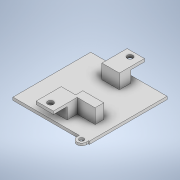
# Autodesk Inventor part: uchwyt2
Saved by Autodesk Inventor 2020.3 (Build 243373000, 373)
## iProperties
Created: 2021-02-11
Part Number: uchwyt2
Material: Ogólny
Document SubType Name: Modeling
Designer: sitar
Density: 1 g/cm^3
Appearance: Domyślna
Author: sitar
Autodesk Inventor part; units mm, degrees
ref_plane "YZ Plane" through (0, 0, 0) normal (1, 0, 0) x (0, 1, 0)
ref_plane "XZ Plane" through (0, 0, 0) normal (0, 1, 0) x (-1, 0, 0)
ref_plane "XY Plane" through (0, 0, 0) normal (0, 0, 1) x (1, 0, 0)
sketch "Szkic1" plane through (0, 0, 0) normal (0, 1, 0) x (-1, 0, 0)
  line L0 (26.7, -27.1) -> (-26.7, -27.1)
  line L1 (-26.7, -27.1) -> (-26.7, 27.1)
  line L2 (-26.7, 27.1) -> (26.7, 27.1)
  line L3 (26.7, 27.1) -> (26.7, -27.1)
  line L4 (26.7, -27.1) -> (-26.7, 27.1) construction
  line L5 (-26.7, -27.1) -> (26.7, 27.1) construction
  point P0 (0, 0)
  dimension "d0" = 53.4
  dimension "d1" = 54.2
  constraints: 12 end point, 2 midpoint, 2 parallel, 1 horizontal, 1 perpendicular
  measures "d0" distance of L1.end L2.end
  measures "d1" distance of L0.end L1.end
extrude "Wyciągnięcie proste1" add sketch "Szkic1" along normal blind 1.6
sketch "Szkic11" plane through (0, 1.6, 0) normal (0, 1, 0) x (1, 0, 0)
  line L0 (-26.7, -27.1) -> (26.7, -27.1) projected
  line L1 (26.7, -27.1) -> (25.9, -27.1)
  line L2 (25.9, -27.1) -> (19.5, -27.1)
  line L3 (19.5, -27.1) -> (19.5, -28.7)
  line L4 (19.5, -28.7) -> (25.9, -28.7)
  line L5 (25.9, -28.7) -> (25.9, -27.1)
  arc A0 (19.5, -28.7) -> (25.9, -28.7) centre (22.7, -28.7) ccw
  point P0 (0, 0)
  dimension "d37" = 0.8
  dimension "d38" = 6.4
  dimension "d39" = 1.6
  dimension "d40" = 3.2
  constraints: 10 end point, 2 parallel, 2 point on circle, 1 centre point, 1 horizontal, 1 perpendicular, 1 point on line
  measures "d37" distance of L0.end L1.end
  measures "d38" distance of L4.end L3.end
  measures "d39" distance of L3.end L2.end
  measures "d40" radius of A0
extrude "Wyciągnięcie proste10" add sketch "Szkic11" against normal blind 1.6
sketch "Szkic12" plane through (0, 1.6, 0) normal (0, 1, 0) x (1, 0, 0)
  arc A0 (19.5, -28.7) -> (25.9, -28.7) centre (22.7, -28.7) ccw projected
  circle A1 centre (22.7, -28.7) radius 1.6
  point P0 (0, 0)
  dimension "d43" = 3.2
  constraints: 1 centre point, 1 coincident
  measures "d43" diameter of A1
extrude "Wyciągnięcie proste11" cut sketch "Szkic12" against normal through all
sketch "Szkic24" plane through (0, 1.6, 0) normal (0, 1, 0) x (1, 0, 0)
  line L0 (11.2, -12.1) -> (11.2, -27.1)
  line L1 (-26.7, -27.1) -> (19.5, -27.1) projected
  line L2 (11.2, -12.1) -> (26.2, -12.1) construction
  line L3 (11.2, -12.1) -> (26.7, -12.1)
  line L4 (26.7, -27.1) -> (26.7, 27.1) projected
  line L5 (11.2, -12.1) -> (26.7, -12.1) construction
  line L6 (4.8, -9.9) -> (17.6, -9.9)
  line L7 (17.6, -9.9) -> (17.6, -14.3)
  line L8 (17.6, -14.3) -> (4.8, -14.3)
  line L9 (4.8, -14.3) -> (4.8, -9.9)
  line L10 (4.8, -9.9) -> (17.6, -14.3) construction
  line L11 (17.6, -9.9) -> (4.8, -14.3) construction
  point P0 (0, 0)
  dimension "d104" = 15
  dimension "d105" = 90
  dimension "d106" = 15.5
  dimension "d107" = 0
  dimension "d108" = 12.8
  dimension "d109" = 4.4
  constraints: 20 end point, 3 horizontal, 3 perpendicular, 2 equal length, 2 midpoint, 2 parallel, 2 point on line
  measures "d104" distance of L0.start L0.end
  measures "d105" angle of L0 L2
  measures "d106" distance of L0.start L3.end
  measures "d107" distance between parallel lines of L3 L5
  measures "d108" distance of L7.end L8.end
  measures "d109" distance of L6.end L7.end
extrude "Wyciągnięcie proste22" cut sketch "Szkic24" against normal through all
sketch "Szkic33" plane through (0, 1.6, 0) normal (0, 1, 0) x (1, 0, 0)
  line L0 (4.8, -14.3) -> (17.6, -14.3) projected
  line L1 (4, 4) -> (4, 25.6) projected
  line L2 (17.6, -14.3) -> (4, -14.3)
  line L3 (4, -14.3) -> (4, -15.1)
  line L4 (4, -15.1) -> (17.6, -15.1)
  line L5 (17.6, -15.1) -> (17.6, -14.3)
  line L6 (4, -15.1) -> (4.8, -15.1)
  line L7 (4.8, -15.1) -> (4.8, -9.1)
  line L8 (4.8, -9.1) -> (4, -9.1)
  line L9 (4, -9.1) -> (4, -15.1)
  line L10 (17.6, -15.1) -> (18.4, -15.1)
  line L11 (18.4, -15.1) -> (18.4, -9.1)
  line L12 (18.4, -9.1) -> (17.6, -9.1)
  line L13 (17.6, -9.1) -> (17.6, -15.1)
  point P0 (0, 0)
  point P1 (4, -21.6)
  point P2 (4, -10)
  point P3 (17.6, -14.3)
  point P4 (4, -10)
  dimension "d139" = 0.8
  dimension "d140" = 6
  dimension "d141" = 0.8
  constraints: 24 end point, 6 parallel, 3 horizontal, 3 perpendicular, 2 point on line
  measures "d139" distance of L3.end L2.end
  measures "d140" distance of L7.end L6.end
  measures "d141" distance of L12.end L11.end
extrude "Wyciągnięcie proste30" add sketch "Szkic33" along normal blind 10
sketch "Szkic34" plane through (0, 1.6, 0) normal (0, 1, 0) x (1, 0, 0)
  line L0 (17.6, -9.9) -> (4.8, -9.9) projected
  line L1 (4.8, -14.3) -> (4.8, -9.1) projected
  line L2 (17.6, -9.9) -> (4.8, -9.9)
  line L3 (4.8, -9.9) -> (4.8, -9.1)
  line L4 (4.8, -9.1) -> (17.6, -9.1)
  line L5 (17.6, -9.1) -> (17.6, -9.9)
  point P0 (0, 0)
  constraints: 8 end point, 2 parallel, 1 horizontal, 1 perpendicular
extrude "Wyciągnięcie proste31" add sketch "Szkic34" along normal blind 2
sketch "Szkic35" plane through (0, 11.6, 0) normal (0, 1, 0) x (1, 0, 0)
  line L0 (4.8, -9.1) -> (4, -9.1) projected
  line L1 (18.4, -15.1) -> (4, -15.1)
  line L2 (4, -15.1) -> (4, -9.1)
  line L3 (4, -9.1) -> (18.4, -9.1)
  line L4 (18.4, -9.1) -> (18.4, -15.1)
  point P0 (0, 0)
  point P1 (4.8, -9.1)
  constraints: 8 end point, 2 parallel, 1 horizontal, 1 perpendicular
extrude "Wyciągnięcie proste32" add sketch "Szkic35" against normal blind 0.8
sketch "Szkic49" plane through (26.7, 0, 27.1) normal (1, 0, 0) x (0, 0, -1)
  line L0 (54.2, 0) -> (54.2, 1.6) projected
  line L1 (0, 0) -> (54.2, 0)
  line L2 (54.2, 0) -> (54.2, 1.6)
  line L3 (54.2, 1.6) -> (0, 1.6)
  line L4 (0, 1.6) -> (0, 0)
  point P0 (27.1, 0)
  constraints: 8 end point, 2 parallel, 1 horizontal, 1 perpendicular
extrude "Wyciągnięcie proste41" cut sketch "Szkic49" against normal blind 0.3
sketch "Szkic50" plane through (-26.7, 0, -27.1) normal (-1, 0, 0) x (0, 0, 1)
  line L0 (0, 1.6) -> (0, 0) projected
  line L1 (0, 0) -> (54.2, 0) projected
  line L2 (0, 1.6) -> (54.2, 1.6)
  line L3 (54.2, 1.6) -> (54.2, 0)
  line L4 (54.2, 0) -> (0, 0)
  line L5 (0, 0) -> (0, 1.6)
  point P0 (27.1, 0)
  constraints: 8 end point, 2 parallel, 1 horizontal, 1 perpendicular
extrude "Wyciągnięcie proste42" cut sketch "Szkic50" against normal blind 0.3
sketch "Szkic57" plane through (0, 0, 0) normal (0, -1, 0) x (1, 0, 0)
  line L0 (-26.4, -27.1) -> (-26.4, 27.1) projected
  line L1 (-26.4, 27.1) -> (26.4, 27.1)
  line L2 (26.4, 27.1) -> (26.4, -27.1)
  line L3 (26.4, -27.1) -> (-26.4, -27.1)
  line L4 (-26.4, -27.1) -> (-26.4, 27.1)
  line L5 (4.8, 14.3) -> (17.6, 14.3) projected
  line L6 (4.8, 9.9) -> (17.6, 9.9) projected
  line L7 (4.8, 14.3) -> (17.6, 14.3)
  line L8 (17.6, 14.3) -> (17.6, 9.9)
  line L9 (17.6, 9.9) -> (4.8, 9.9)
  line L10 (4.8, 9.9) -> (4.8, 14.3)
  point P0 (0, 0)
  point P1 (17.6, 14.3)
  constraints: 16 end point, 4 parallel, 2 horizontal, 2 perpendicular
extrude "Wyciągnięcie proste48" add sketch "Szkic57" along normal blind 0.4
sketch "Szkic62" plane through (26.4, 1.6, -27.1) normal (0, 0, -1) x (-1, 0, 0)
  line L0 (52.8, 0) -> (52.8, -2) projected
  line L1 (52.8, -2) -> (0, -2)
  line L2 (0, -2) -> (0, 0)
  line L3 (0, 0) -> (52.8, 0)
  line L4 (52.8, 0) -> (52.8, -2)
  point P0 (26.4, -1.6)
  constraints: 8 end point, 2 parallel, 1 horizontal, 1 perpendicular
extrude "Wyciągnięcie proste52" cut sketch "Szkic62" against normal blind 0.4
sketch "Szkic63" plane through (0, 1.6, 0) normal (0, 1, 0) x (1, 0, 0)
  line L0 (0, 0) -> (0, 27.5)
  line L1 (0, 0) -> (27.5, 0) construction
  circle A0 centre (0, 27.5) radius 2
  line L2 (0, 0) -> (0, -27.5)
  line L3 (0, 0) -> (27.5, 0) construction
  circle A1 centre (0, -27.5) radius 2
  dimension "d235" = 27.5
  dimension "d236" = 90
  dimension "d237" = 4
  dimension "d238" = 27.5
  dimension "d239" = 90
  dimension "d240" = 4
  constraints: 8 end point, 2 centre point, 2 coincident, 2 horizontal, 2 perpendicular, 2 vertical
  measures "d235" distance of L0.start L0.end
  measures "d236" angle of L1 L0
  measures "d237" diameter of A0
  measures "d238" distance of L0.start L2.end
  measures "d239" angle of L2 L3
  measures "d240" diameter of A1
sketch "Szkic64" plane through (0, 1.6, 0) normal (0, 1, 0) x (1, 0, 0)
  line L0 (26.4, 26.7) -> (-26.4, 26.7) projected
  line L1 (0, 26.7) -> (0, 25.1)
  line L2 (0, 25.1) -> (-4, 25.1)
  line L3 (-4, 25.1) -> (-4, 18.7)
  line L4 (-4, 18.7) -> (0, 18.7)
  line L5 (0, 18.7) -> (0, 25.1)
  point P0 (0, 0)
  dimension "d241" = 1.6
  dimension "d242" = 4
  dimension "d243" = 6.4
  constraints: 10 end point, 2 parallel, 1 horizontal, 1 midpoint, 1 perpendicular, 1 vertical
  measures "d241" distance of L1.start L1.end
  measures "d242" distance of L4.end L3.end
  measures "d243" distance of L3.end L2.end
extrude "Wyciągnięcie proste53" add sketch "Szkic64" along normal blind 8
mirror "Odbij11" about plane through (0, 0, 0) normal (1, 0, 0) of "Wyciągnięcie proste53"
sketch "Szkic65" plane through (0, 9.6, 0) normal (0, 1, 0) x (1, 0, 0)
  line L0 (-4, 25.1) -> (4, 25.1) projected
  line L1 (-4, 25.1) -> (4, 25.1)
  line L2 (4, 25.1) -> (4, 31.5)
  line L3 (4, 31.5) -> (-4, 31.5)
  line L4 (-4, 31.5) -> (-4, 25.1)
  point P0 (0, 0)
  dimension "d246" = 6.4
  constraints: 8 end point, 2 parallel, 1 horizontal, 1 perpendicular
  measures "d246" distance of L2.end L1.end
extrude "Wyciągnięcie proste54" add sketch "Szkic65" along normal blind 2
mirror "Odbij12" about plane through (0, 0, 0) normal (0, 0, 1) of "Wyciągnięcie proste53", "Odbij11", "Wyciągnięcie proste54"
extrude "Wyciągnięcie proste55" cut sketch "Szkic63" along normal through all
sketch "Szkic66" plane through (0, 9.6, 0) normal (0, 1, 0) x (1, 0, 0)
  line L0 (-4, 18.7) -> (-4, 25.1) projected
  line L1 (-4, 25.1) -> (4, 25.1) projected
  line L2 (-4, 18.7) -> (4, 18.7)
  line L3 (4, 18.7) -> (4, 25.1)
  line L4 (4, 25.1) -> (-4, 25.1)
  line L5 (-4, 25.1) -> (-4, 18.7)
  line L6 (-4, -25.1) -> (-4, -18.7) projected
  line L7 (-4, -25.1) -> (4, -25.1) projected
  line L8 (-4, -18.7) -> (4, -18.7)
  line L9 (4, -18.7) -> (4, -25.1)
  line L10 (4, -25.1) -> (-4, -25.1)
  line L11 (-4, -25.1) -> (-4, -18.7)
  point P0 (0, 0)
  constraints: 16 end point, 4 parallel, 2 horizontal, 2 perpendicular
extrude "Wyciągnięcie proste56" add sketch "Szkic66" along normal blind 2
sketch "Szkic67" plane through (4, 1.6, -25.1) normal (0, 0, -1) x (-1, 0, 0)
  line L0 (0, 8) -> (8, 8) projected
  line L1 (8, 0) -> (0, 0) projected
  line L2 (8, 8) -> (0, 8)
  line L3 (0, 8) -> (0, 0)
  line L4 (0, 0) -> (8, 0)
  line L5 (8, 0) -> (8, 8)
  point P0 (4, -1.6)
  constraints: 8 end point, 2 parallel, 1 horizontal, 1 perpendicular
extrude "Wyciągnięcie proste57" cut sketch "Szkic67" against normal blind 3
sketch "Szkic68" plane through (-4, 1.6, -18.7) normal (0, 0, 1) x (1, 0, 0)
  line L0 (8, 0) -> (8, 10) projected
  line L1 (8, 0) -> (0, 0) projected
  line L2 (8, 10) -> (0, 10)
  line L3 (0, 10) -> (0, 0)
  line L4 (0, 0) -> (8, 0)
  line L5 (8, 0) -> (8, 10)
  point P0 (4, -1.6)
  constraints: 8 end point, 2 parallel, 1 horizontal, 1 perpendicular
extrude "Wyciągnięcie proste58" add sketch "Szkic68" along normal blind 4.6
sketch "Szkic69" plane through (-4, 9.6, -31.5) normal (-1, 0, 0) x (0, 0, 1)
  line L0 (17.4, 2) -> (17.4, -8) projected
  line L1 (17.4, 2) -> (17.4, -8)
  line L2 (9.4, -8) -> (17.4, -8) projected
  line L3 (17.4, -8) -> (9.4, -8)
  line L4 (9.4, -8) -> (9.4, 0) projected
  line L5 (9.4, -8) -> (9.4, 0)
  line L6 (0, 0) -> (0, 2) projected
  line L7 (9.4, 0) -> (0, 0)
  line L8 (0, 0) -> (0, 2)
  line L9 (0, 2) -> (17.4, 2) projected
  line L10 (0, 2) -> (17.4, 2)
  point P0 (31.5, -9.6)
  constraints: 12 end point, 3 collinear, 2 perpendicular, 1 vertical
extrude "Wyciągnięcie proste59" add sketch "Szkic69" along normal blind 2
mirror "Odbij13" about plane through (0, 0, 0) normal (1, 0, 0) of "Wyciągnięcie proste59"
mirror "Odbij14" about plane through (0, 0, 0) normal (0, 0, 1) of "Wyciągnięcie proste56", "Wyciągnięcie proste57", "Wyciągnięcie proste58", "Wyciągnięcie proste59", "Odbij13"
sketch "Szkic70" plane through (4.8, 1.6, 14.3) normal (0, -1, 0) x (1, 0, 0)
  line L0 (0, -0.2) -> (1.2, -0.2) projected
  line L1 (1.2, -0.2) -> (0, -0.2)
  line L2 (0, -0.2) -> (0, 0)
  line L3 (0, 0) -> (1.2, 0)
  line L4 (1.2, 0) -> (1.2, -0.2)
  point P0 (-4.8, -14.3)
  constraints: 8 end point, 2 parallel, 1 horizontal, 1 perpendicular
extrude "Wyciągnięcie proste60" cut sketch "Szkic70" against normal up to surface (9.2 mm away)
